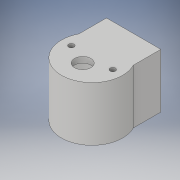
# Autodesk Inventor part: Suspension Bracket Mount
Saved by Autodesk Inventor 2018.2 (Build 222227000, 227)
## iProperties
Created: 2018-02-09
Part Number: Suspension Bracket Mount
Material: Generic
Document SubType Name: Modeling
Designer: MIABo
Density: 1 g/cm^3
Appearance: Default
Author: MIABo
Autodesk Inventor part; units mm, degrees
ref_plane "YZ Plane" through (0, 0, 0) normal (1, 0, 0) x (0, 1, 0)
ref_plane "XZ Plane" through (0, 0, 0) normal (0, 1, 0) x (-1, 0, 0)
ref_plane "XY Plane" through (0, 0, 0) normal (0, 0, 1) x (1, 0, 0)
ref_plane "Work Plane2" through (0, 0, 0) normal (0, 0, 1) x (1, 0, 0)
sketch "Sketch1" plane through (0, 0, 0) normal (0, 0, 1) x (1, 0, 0)
  line L0 (29.5603, 0.0547) -> (16.8603, 0.0547)
  line L1 (16.8603, 0.0547) -> (16.8603, 40.6947)
  line L2 (16.8603, 40.6947) -> (29.5603, 40.6947)
  line L3 (29.5603, 40.6947) -> (29.5603, 0.0547)
  point P0 (0, 0)
  dimension "d0" = 12.7
  dimension "d1" = 40.64
  constraints: 8 end point, 2 parallel, 1 horizontal, 1 perpendicular
  measures "d0" distance of L1.end L2.end
  measures "d1" distance of L0.end L1.end
extrude "Extrusion1" add sketch "Sketch1" along normal blind 12.7
sketch "Sketch2" plane through (16.8603, 40.6947, 0) normal (0, 1, 0) x (1, 0, 0)
  circle A0 centre (6.35, -31.115) radius 18.415
  line L0 (12.7, -12.7) -> (0, -12.7) projected
  line L1 (0, 0) -> (0, -12.7) projected
  circle A1 centre (6.35, -31.115) radius 22.86
  point P0 (-16.8603, 0)
  point P1 (6.35, -12.7)
  dimension "d4" = 36.83
  dimension "d6" = 6.35
  dimension "d7" = 45.72
  constraints: 1 centre point, 1 coincident, 1 midpoint, 1 vertical alignment, 2 other
  measures "d6" distance from line of point (6.35, -31.115) L1
  measures "d7" diameter of A1
extrude "Extrusion2" add sketch "Sketch2" against normal blind 40.64
sketch "Sketch3" plane through (16.8603, 40.6947, 0) normal (0, 1, 0) x (1, 0, 0)
  circle A0 centre (6.35, -31.115) radius 18.415
  circle A1 centre (6.35, -31.115) radius 18.415 projected
  circle A2 centre (21.844, -31.115) radius 1.9939
  circle A3 centre (-9.144, -31.115) radius 1.9939
  circle A4 centre (6.35, -38.1254) radius 6.096
  point P0 (-16.8603, 0)
  point P1 (2.6162, -31.115)
  dimension "d10" = 36.83
  dimension "d21" = 3.9878
  dimension "d22" = 3.9878
  dimension "d23" = 30.988
  dimension "d27" = 12.192
  dimension "d28" = 7.0104
  constraints: 4 centre point, 1 coincident, 1 concentric, 1 vertical alignment
  measures "d10" diameter of A0
  measures "d21" diameter of A2
  measures "d22" diameter of A3
  measures "d23" distance of A3.centre A2.centre
  measures "d27" diameter of A4
  measures "d28" distance of A4.centre A1.centre
extrude "Extrusion3" add sketch "Sketch3" against normal blind 4.318
sketch "Sketch6" plane through (0, 0, 0) normal (0, 0, -1) x (-1, 0, 0)
  line L0 (-16.8603, 0.0547) -> (-2.8903, 0.0547)
  line L1 (-2.8903, 0.0547) -> (-2.8903, 40.6947)
  line L2 (-2.8903, 40.6947) -> (-16.8603, 40.6947)
  line L3 (-16.8603, 40.6947) -> (-16.8603, 0.0547)
  point P0 (0, 0)
  dimension "d36" = 13.97
  dimension "d37" = 40.64
  constraints: 8 end point, 2 parallel, 1 horizontal, 1 perpendicular
  measures "d36" distance of L2.end L1.end
  measures "d37" distance of L0.end L1.end
extrude "Extrusion4" add sketch "Sketch6" against normal up to next
sketch "Sketch7" plane through (0, 0, 0) normal (0, 0, -1) x (-1, 0, 0)
  line L0 (-29.5603, 40.6947) -> (-29.5603, 0.0547) projected
  line L1 (-46.0703, 40.6947) -> (-0.3503, 40.6947) projected
  line L2 (-29.5603, 0.0547) -> (-43.5303, 0.0547)
  line L3 (-43.5303, 0.0547) -> (-43.5303, 40.6947)
  line L4 (-43.5303, 40.6947) -> (-29.5603, 40.6947)
  line L5 (-29.5603, 40.6947) -> (-29.5603, 0.0547)
  point P0 (0, 0)
  point P1 (-2.8903, 40.6947)
  dimension "d40" = 13.97
  constraints: 8 end point, 2 parallel, 1 horizontal, 1 perpendicular, 1 point on line
  measures "d40" distance of L3.end L4.end
extrude "Extrusion5" add sketch "Sketch7" against normal up to next
body "Solid1"
